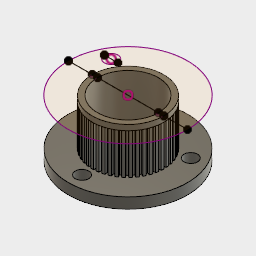
Slip Joint Gear v2 (Autodesk Fusion 360 design; units mm, degrees)
Autodesk Fusion 360 part; units mm, degrees
sketch "Sketch1" plane through (0, 0, 0) normal (0, 1, 0) x (1, 0, 0)
  circle A0 centre (0, 0) radius 22
  circle A1 centre (0, 0) radius 11.25
  line L0 (-0.0017, -22) -> (-0.0017, -19.5)
  circle A2 centre (-0.0017, -17) radius 2.5
  circle A3 centre (14.7233, 8.4986) radius 2.5
  circle A4 centre (-14.7216, 8.5014) radius 2.5
  dimension "d1" = 44
  dimension "d2" = 22.5
  dimension "d3" = 2.5
  dimension "d4" = 5
  dimension "d6" = 360
  measures "d1" diameter of A0
  measures "d2" diameter of A1
  measures "d3" distance of L0.start L0.end
  measures "d4" diameter of A2
extrude "Extrude1" add sketch "Sketch1" along normal blind 4
sketch "Sketch2" plane through (0, 4, 0) normal (0, 1, 0) x (-1, 0, 0)
  circle A0 centre (0, 0) radius 11.25
  circle A1 centre (14.7216, -8.5014) radius 2.5
  circle A2 centre (-14.7233, -8.4986) radius 2.5
  circle A3 centre (0.0017, 17) radius 2.5
  circle A4 centre (0, 0) radius 22
  circle A5 centre (0, 0) radius 12.25
  line L0 (0.0002, 13.25) -> (-0.5, 13.25)
  line L1 (-0.5, 13.25) -> (0.0002, 13.25)
  line L2 (0.0002, 13.25) -> (0.5, 13.25)
  line L3 (0.5, 13.25) -> (0.5, 12.2398)
  line L4 (-0.5, 13.25) -> (-0.5, 12.2398)
  line L5 (-2.3392, 13.0515) -> (-2.1986, 12.0511)
  line L6 (-1.8438, 13.1211) -> (-2.3392, 13.0515)
  line L7 (-1.8438, 13.1211) -> (-1.3489, 13.1906)
  line L8 (-1.3489, 13.1906) -> (-1.2083, 12.1903)
  line L9 (-4.1328, 12.5989) -> (-3.8544, 11.6278)
  line L10 (-3.652, 12.7368) -> (-4.1328, 12.5989)
  line L11 (-3.652, 12.7368) -> (-3.1716, 12.8745)
  line L12 (-3.1716, 12.8745) -> (-2.8931, 11.9035)
  line L13 (-5.846, 11.9011) -> (-5.4351, 10.9782)
  line L14 (-5.3891, 12.1046) -> (-5.846, 11.9011)
  line L15 (-5.3891, 12.1046) -> (-4.9325, 12.3078)
  line L16 (-4.9325, 12.3078) -> (-4.5216, 11.385)
  line L17 (-7.4455, 10.9717) -> (-6.9101, 10.115)
  line L18 (-7.0213, 11.2367) -> (-7.4455, 10.9717)
  line L19 (-7.0213, 11.2367) -> (-6.5974, 11.5016)
  line L20 (-6.5974, 11.5016) -> (-6.0621, 10.6449)
  line L21 (-8.9, 9.8287) -> (-8.2506, 9.0548)
  line L22 (-8.5168, 10.1502) -> (-8.9, 9.8287)
  line L23 (-8.5168, 10.1502) -> (-8.1339, 10.4715)
  line L24 (-8.1339, 10.4715) -> (-7.4846, 9.6976)
  line L25 (-10.1812, 8.4944) -> (-9.4305, 7.8184)
  line L26 (-9.8465, 8.8661) -> (-10.1812, 8.4944)
  line L27 (-9.8465, 8.8661) -> (-9.5121, 9.2376)
  line L28 (-9.5121, 9.2376) -> (-8.7614, 8.5616)
  line L29 (-11.2643, 6.9948) -> (-10.4268, 6.4299)
  line L30 (-10.9846, 7.4095) -> (-11.2643, 6.9948)
  line L31 (-10.9846, 7.4095) -> (-10.7052, 7.8238)
  line L32 (-10.7052, 7.8238) -> (-9.8677, 7.2589)
  line L33 (-12.1282, 5.359) -> (-11.2202, 4.9162)
  line L34 (-11.9089, 5.8086) -> (-12.1282, 5.359)
  line L35 (-11.9089, 5.8086) -> (-11.6898, 6.2578)
  line L36 (-11.6898, 6.2578) -> (-10.7819, 5.815)
  line L37 (-12.756, 3.6189) -> (-11.7952, 3.3068)
  line L38 (-12.6014, 4.0947) -> (-12.756, 3.6189)
  line L39 (-12.6014, 4.0947) -> (-12.447, 4.57)
  line L40 (-12.447, 4.57) -> (-11.4862, 4.2578)
  line L41 (-13.1355, 1.8084) -> (-12.1407, 1.633)
  line L42 (-13.0487, 2.301) -> (-13.1355, 1.8084)
  line L43 (-13.0487, 2.301) -> (-12.9619, 2.7932)
  line L44 (-12.9619, 2.7932) -> (-11.967, 2.6178)
  line L45 (-13.2594, -0.0373) -> (-12.2498, -0.0725)
  line L46 (-13.2419, 0.4626) -> (-13.2594, -0.0373)
  line L47 (-13.2419, 0.4626) -> (-13.2245, 0.9621)
  line L48 (-13.2245, 0.9621) -> (-12.2149, 0.9269)
  line L49 (-13.1252, -1.8823) -> (-12.1205, -1.7767)
  line L50 (-13.1774, -1.3848) -> (-13.1252, -1.8823)
  line L51 (-13.1774, -1.3848) -> (-13.2297, -0.8877)
  line L52 (-13.2297, -0.8877) -> (-12.225, -0.7821)
  line L53 (-12.7355, -3.6906) -> (-11.7553, -3.4462)
  line L54 (-12.8565, -3.2053) -> (-12.7355, -3.6906)
  line L55 (-12.8565, -3.2053) -> (-12.9774, -2.7203)
  line L56 (-12.9774, -2.7203) -> (-11.9972, -2.4759)
  line L57 (-12.0979, -5.4271) -> (-11.1612, -5.0487)
  line L58 (-12.2853, -4.9634) -> (-12.0979, -5.4271)
  line L59 (-12.2853, -4.9634) -> (-12.4725, -4.4999)
  line L60 (-12.4725, -4.4999) -> (-11.5358, -4.1215)
  line L61 (-11.2248, -7.058) -> (-10.35, -6.5529)
  line L62 (-11.4749, -6.6248) -> (-11.2248, -7.058)
  line L63 (-11.4749, -6.6248) -> (-11.7248, -6.192)
  line L64 (-11.7248, -6.192) -> (-10.85, -5.6869)
  line L65 (-10.1333, -8.5515) -> (-9.3373, -7.9296)
  line L66 (-10.4413, -8.1574) -> (-10.1333, -8.5515)
  line L67 (-10.4413, -8.1574) -> (-10.749, -7.7635)
  line L68 (-10.749, -7.7635) -> (-9.9529, -7.1416)
  line L69 (-8.8446, -9.8786) -> (-8.1428, -9.1519)
  line L70 (-9.2044, -9.5311) -> (-8.8446, -9.8786)
  line L71 (-9.2044, -9.5311) -> (-9.5639, -9.1839)
  line L72 (-9.5639, -9.1839) -> (-8.8621, -8.4572)
  line L73 (-7.3836, -11.0134) -> (-6.7899, -10.1961)
  line L74 (-7.7883, -10.7194) -> (-7.3836, -11.0134)
  line L75 (-7.7883, -10.7194) -> (-8.1927, -10.4256)
  line L76 (-8.1927, -10.4256) -> (-7.5989, -9.6083)
  line L77 (-5.779, -11.9338) -> (-5.3048, -11.0418)
  line L78 (-6.2207, -11.699) -> (-5.779, -11.9338)
  line L79 (-6.2207, -11.699) -> (-6.662, -11.4643)
  line L80 (-6.662, -11.4643) -> (-6.1877, -10.5724)
  line L81 (-4.0619, -12.6219) -> (-3.7164, -11.6727)
  line L82 (-4.532, -12.4509) -> (-4.0619, -12.6219)
  line L83 (-4.532, -12.4509) -> (-5.0016, -12.2799)
  line L84 (-5.0016, -12.2799) -> (-4.6561, -11.3306)
  line L85 (-2.2658, -13.0644) -> (-2.0557, -12.0763)
  line L86 (-2.755, -12.9604) -> (-2.2658, -13.0644)
  line L87 (-2.755, -12.9604) -> (-3.2439, -12.8565)
  line L88 (-3.2439, -12.8565) -> (-3.0339, -11.8684)
  line L89 (-0.4255, -13.2526) -> (-0.355, -12.2449)
  line L90 (-0.9245, -13.2177) -> (-0.4255, -13.2526)
  line L91 (-0.9245, -13.2177) -> (-1.4231, -13.1828)
  line L92 (-1.4231, -13.1828) -> (-1.3526, -12.1751)
  line L93 (1.4231, -13.1828) -> (1.3526, -12.1751)
  line L94 (0.9241, -13.2177) -> (1.4231, -13.1828)
  line L95 (0.9241, -13.2177) -> (0.4255, -13.2526)
  line L96 (0.4255, -13.2526) -> (0.355, -12.2449)
  line L97 (3.2439, -12.8565) -> (3.0339, -11.8684)
  line L98 (2.7546, -12.9605) -> (3.2439, -12.8565)
  line L99 (2.7546, -12.9605) -> (2.2658, -13.0644)
  line L100 (2.2658, -13.0644) -> (2.0557, -12.0763)
  line L101 (5.0016, -12.2799) -> (4.6561, -11.3306)
  line L102 (4.5316, -12.451) -> (5.0016, -12.2799)
  line L103 (4.5316, -12.451) -> (4.0619, -12.6219)
  line L104 (4.0619, -12.6219) -> (3.7164, -11.6727)
  line L105 (6.662, -11.4643) -> (6.1877, -10.5724)
  line L106 (6.2203, -11.6992) -> (6.662, -11.4643)
  line L107 (6.2203, -11.6992) -> (5.779, -11.9338)
  line L108 (5.779, -11.9338) -> (5.3048, -11.0418)
  line L109 (8.1927, -10.4256) -> (7.5989, -9.6083)
  line L110 (7.788, -10.7196) -> (8.1927, -10.4256)
  line L111 (7.788, -10.7196) -> (7.3836, -11.0134)
  line L112 (7.3836, -11.0134) -> (6.7899, -10.1961)
  line L113 (9.5639, -9.1839) -> (8.8621, -8.4572)
  line L114 (9.2041, -9.5314) -> (9.5639, -9.1839)
  line L115 (9.2041, -9.5314) -> (8.8446, -9.8786)
  line L116 (8.8446, -9.8786) -> (8.1428, -9.1519)
  line L117 (10.749, -7.7635) -> (9.9529, -7.1416)
  line L118 (10.441, -8.1577) -> (10.749, -7.7635)
  line L119 (10.441, -8.1577) -> (10.1333, -8.5515)
  line L120 (10.1333, -8.5515) -> (9.3373, -7.9296)
  line L121 (11.7248, -6.192) -> (10.85, -5.6869)
  line L122 (11.4747, -6.6252) -> (11.7248, -6.192)
  line L123 (11.4747, -6.6252) -> (11.2248, -7.058)
  line L124 (11.2248, -7.058) -> (10.35, -6.5529)
  line L125 (12.4725, -4.4999) -> (11.5358, -4.1215)
  line L126 (12.2851, -4.9637) -> (12.4725, -4.4999)
  line L127 (12.2851, -4.9637) -> (12.0979, -5.4271)
  line L128 (12.0979, -5.4271) -> (11.1612, -5.0487)
  line L129 (12.9774, -2.7203) -> (11.9972, -2.4759)
  line L130 (12.8564, -3.2057) -> (12.9774, -2.7203)
  line L131 (12.8564, -3.2057) -> (12.7355, -3.6906)
  line L132 (12.7355, -3.6906) -> (11.7553, -3.4462)
  line L133 (13.2297, -0.8877) -> (12.225, -0.7821)
  line L134 (13.1774, -1.3852) -> (13.2297, -0.8877)
  line L135 (13.1774, -1.3852) -> (13.1252, -1.8823)
  line L136 (13.1252, -1.8823) -> (12.1205, -1.7767)
  line L137 (13.2245, 0.9621) -> (12.2149, 0.9269)
  line L138 (13.2419, 0.4622) -> (13.2245, 0.9621)
  line L139 (13.2419, 0.4622) -> (13.2594, -0.0373)
  line L140 (13.2594, -0.0373) -> (12.2498, -0.0725)
  line L141 (12.9619, 2.7932) -> (11.967, 2.6178)
  line L142 (13.0487, 2.3006) -> (12.9619, 2.7932)
  line L143 (13.0487, 2.3006) -> (13.1355, 1.8084)
  line L144 (13.1355, 1.8084) -> (12.1407, 1.633)
  line L145 (12.447, 4.57) -> (11.4862, 4.2578)
  line L146 (12.6016, 4.0943) -> (12.447, 4.57)
  line L147 (12.6016, 4.0943) -> (12.756, 3.6189)
  line L148 (12.756, 3.6189) -> (11.7952, 3.3068)
  line L149 (11.6898, 6.2578) -> (10.7819, 5.815)
  line L150 (11.9091, 5.8082) -> (11.6898, 6.2578)
  line L151 (11.9091, 5.8082) -> (12.1282, 5.359)
  line L152 (12.1282, 5.359) -> (11.2202, 4.9162)
  line L153 (10.7052, 7.8238) -> (9.8677, 7.2589)
  line L154 (10.9849, 7.4091) -> (10.7052, 7.8238)
  line L155 (10.9849, 7.4091) -> (11.2643, 6.9948)
  line L156 (11.2643, 6.9948) -> (10.4268, 6.4299)
  line L157 (9.5121, 9.2376) -> (8.7614, 8.5616)
  line L158 (9.8468, 8.8658) -> (9.5121, 9.2376)
  line L159 (9.8468, 8.8658) -> (10.1812, 8.4944)
  line L160 (10.1812, 8.4944) -> (9.4305, 7.8184)
  line L161 (8.1339, 10.4715) -> (7.4846, 9.6976)
  line L162 (8.5171, 10.15) -> (8.1339, 10.4715)
  line L163 (8.5171, 10.15) -> (8.9, 9.8287)
  line L164 (8.9, 9.8287) -> (8.2506, 9.0548)
  line L165 (6.5974, 11.5016) -> (6.0621, 10.6449)
  line L166 (7.0216, 11.2365) -> (6.5974, 11.5016)
  line L167 (7.0216, 11.2365) -> (7.4455, 10.9717)
  line L168 (7.4455, 10.9717) -> (6.9101, 10.115)
  line L169 (4.9325, 12.3078) -> (4.5216, 11.385)
  line L170 (5.3894, 12.1044) -> (4.9325, 12.3078)
  line L171 (5.3894, 12.1044) -> (5.846, 11.9011)
  line L172 (5.846, 11.9011) -> (5.4351, 10.9782)
  line L173 (3.1716, 12.8745) -> (2.8931, 11.9035)
  line L174 (3.6524, 12.7367) -> (3.1716, 12.8745)
  line L175 (3.6524, 12.7367) -> (4.1328, 12.5989)
  line L176 (4.1328, 12.5989) -> (3.8544, 11.6278)
  line L177 (1.3489, 13.1906) -> (1.2083, 12.1903)
  line L178 (1.8442, 13.121) -> (1.3489, 13.1906)
  line L179 (1.8442, 13.121) -> (2.3392, 13.0515)
  line L180 (2.3392, 13.0515) -> (2.1986, 12.0511)
  dimension "d9" = 24.5
  dimension "d12" = 360
  measures "d9" diameter of A5
extrude "Extrude2" add sketch "Sketch2" along normal blind 15 contours A5 | A5 L137 L138 L139 L140 | A5 L141 L142 L143 L144 | A5 L133 L134 L135 L136 | A5 L145 L146 L147 L148 | A5 L129 L130 L131 L132 | A5 L149 L150 L151 L152 | A5 L125 L126 L127 L128 | A5 L153 L154 L155 L156 | A5 L121 L122 L123 L124 | A5 L157 L158 L159 L160 | A5 L117 L118 L119 L120 | A5 L161 L162 L163 L164 | A5 L113 L114 L115 L116 | A5 L165 L166 L167 L168 | A5 L109 L110 L111 L112 | A5 L169 L170 L171 L172 | A5 L105 L106 L107 L108 | A5 L173 L174 L175 L176 | A5 L101 L102 L103 L104 | A5 L177 L178 L179 L180 | A5 L97 L98 L99 L100 | A5 L0 L1 L2 L3 L4 | A5 L93 L94 L95 L96 | A5 L5 L6 L7 L8 | A5 L89 L90 L91 L92 | A5 L9 L10 L11 L12 | A5 L85 L86 L87 L88 | A5 L13 L14 L15 L16 | A5 L81 L82 L83 L84 | A5 L17 L18 L19 L20 | A5 L77 L78 L79 L80 | A5 L21 L22 L23 L24 | A5 L73 L74 L75 L76 | A5 L25 L26 L27 L28 | A5 L69 L70 L71 L72 | A5 L29 L30 L31 L32 | A5 L65 L66 L67 L68 | A5 L33 L34 L35 L36 | A5 L61 L62 L63 L64 | A5 L37 L38 L39 L40 | A5 L57 L58 L59 L60 | A5 L41 L42 L43 L44 | A5 L53 L54 L55 L56 | A5 L45 L46 L47 L48 | A5 L49 L50 L51 L52
sketch "Sketch3" plane through (0, 19, 0) normal (0, 1, 0) x (-1, 0, 0)
  circle A0 centre (0, 0) radius 11.25
  line L0 (2.3392, 13.0515) -> (1.3489, 13.1906)
  line L1 (1.3489, 13.1906) -> (1.2083, 12.1903)
  arc A1 (1.2083, 12.1903) -> (0.5, 12.2398) centre (0, 0) ccw
  line L2 (0.5, 12.2398) -> (0.5, 13.25)
  line L3 (0.5, 13.25) -> (-0.5, 13.25)
  line L4 (-0.5, 13.25) -> (-0.5, 12.2398)
  arc A2 (-0.5, 12.2398) -> (-1.2083, 12.1903) centre (0, 0) ccw
  line L5 (-1.2083, 12.1903) -> (-1.3489, 13.1906)
  line L6 (-1.3489, 13.1906) -> (-2.3392, 13.0515)
  line L7 (-2.3392, 13.0515) -> (-2.1986, 12.0511)
  arc A3 (-2.1986, 12.0511) -> (-2.8931, 11.9035) centre (0, 0) ccw
  line L8 (-2.8931, 11.9035) -> (-3.1716, 12.8745)
  line L9 (-3.1716, 12.8745) -> (-4.1328, 12.5989)
  line L10 (-4.1328, 12.5989) -> (-3.8544, 11.6278)
  arc A4 (-3.8544, 11.6278) -> (-4.5216, 11.385) centre (0, 0) ccw
  line L11 (-4.5216, 11.385) -> (-4.9325, 12.3078)
  line L12 (-4.9325, 12.3078) -> (-5.846, 11.9011)
  line L13 (-5.846, 11.9011) -> (-5.4351, 10.9782)
  arc A5 (-5.4351, 10.9782) -> (-6.0621, 10.6449) centre (0, 0) ccw
  line L14 (-6.0621, 10.6449) -> (-6.5974, 11.5016)
  line L15 (-6.5974, 11.5016) -> (-7.4455, 10.9717)
  line L16 (-7.4455, 10.9717) -> (-6.9101, 10.115)
  arc A6 (-6.9101, 10.115) -> (-7.4846, 9.6976) centre (0, 0) ccw
  line L17 (-7.4846, 9.6976) -> (-8.1339, 10.4715)
  line L18 (-8.1339, 10.4715) -> (-8.9, 9.8287)
  line L19 (-8.9, 9.8287) -> (-8.2506, 9.0548)
  arc A7 (-8.2506, 9.0548) -> (-8.7614, 8.5616) centre (0, 0) ccw
  line L20 (-8.7614, 8.5616) -> (-9.5121, 9.2376)
  line L21 (-9.5121, 9.2376) -> (-10.1812, 8.4944)
  line L22 (-10.1812, 8.4944) -> (-9.4305, 7.8184)
  arc A8 (-9.4305, 7.8184) -> (-9.8677, 7.2589) centre (0, 0) ccw
  line L23 (-9.8677, 7.2589) -> (-10.7052, 7.8238)
  line L24 (-10.7052, 7.8238) -> (-11.2643, 6.9948)
  line L25 (-11.2643, 6.9948) -> (-10.4268, 6.4299)
  arc A9 (-10.4268, 6.4299) -> (-10.7819, 5.815) centre (0, 0) ccw
  line L26 (-10.7819, 5.815) -> (-11.6898, 6.2578)
  line L27 (-11.6898, 6.2578) -> (-12.1282, 5.359)
  line L28 (-12.1282, 5.359) -> (-11.2202, 4.9162)
  arc A10 (-11.2202, 4.9162) -> (-11.4862, 4.2578) centre (0, 0) ccw
  line L29 (-11.4862, 4.2578) -> (-12.447, 4.57)
  line L30 (-12.447, 4.57) -> (-12.756, 3.6189)
  line L31 (-12.756, 3.6189) -> (-11.7952, 3.3068)
  arc A11 (-11.7952, 3.3068) -> (-11.967, 2.6178) centre (0, 0) ccw
  line L32 (-11.967, 2.6178) -> (-12.9619, 2.7932)
  line L33 (-12.9619, 2.7932) -> (-13.1355, 1.8084)
  line L34 (-13.1355, 1.8084) -> (-12.1407, 1.633)
  arc A12 (-12.1407, 1.633) -> (-12.2149, 0.9269) centre (0, 0) ccw
  line L35 (-12.2149, 0.9269) -> (-13.2245, 0.9621)
  line L36 (-13.2245, 0.9621) -> (-13.2594, -0.0373)
  line L37 (-13.2594, -0.0373) -> (-12.2498, -0.0725)
  arc A13 (-12.2498, -0.0725) -> (-12.225, -0.7821) centre (0, 0) ccw
  line L38 (-12.225, -0.7821) -> (-13.2297, -0.8877)
  line L39 (-13.2297, -0.8877) -> (-13.1252, -1.8823)
  line L40 (-13.1252, -1.8823) -> (-12.1205, -1.7767)
  arc A14 (-12.1205, -1.7767) -> (-11.9972, -2.4759) centre (0, 0) ccw
  line L41 (-11.9972, -2.4759) -> (-12.9774, -2.7203)
  line L42 (-12.9774, -2.7203) -> (-12.7355, -3.6906)
  line L43 (-12.7355, -3.6906) -> (-11.7553, -3.4462)
  arc A15 (-11.7553, -3.4462) -> (-11.5358, -4.1215) centre (0, 0) ccw
  line L44 (-11.5358, -4.1215) -> (-12.4725, -4.4999)
  line L45 (-12.4725, -4.4999) -> (-12.0979, -5.4271)
  line L46 (-12.0979, -5.4271) -> (-11.1612, -5.0487)
  arc A16 (-11.1612, -5.0487) -> (-10.85, -5.6869) centre (0, 0) ccw
  line L47 (-10.85, -5.6869) -> (-11.7248, -6.192)
  line L48 (-11.7248, -6.192) -> (-11.2248, -7.058)
  line L49 (-11.2248, -7.058) -> (-10.35, -6.5529)
  arc A17 (-10.35, -6.5529) -> (-9.9529, -7.1416) centre (0, 0) ccw
  line L50 (-9.9529, -7.1416) -> (-10.749, -7.7635)
  line L51 (-10.749, -7.7635) -> (-10.1333, -8.5515)
  line L52 (-10.1333, -8.5515) -> (-9.3373, -7.9296)
  arc A18 (-9.3373, -7.9296) -> (-8.8621, -8.4572) centre (0, 0) ccw
  line L53 (-8.8621, -8.4572) -> (-9.5639, -9.1839)
  line L54 (-9.5639, -9.1839) -> (-8.8446, -9.8786)
  line L55 (-8.8446, -9.8786) -> (-8.1428, -9.1519)
  arc A19 (-8.1428, -9.1519) -> (-7.5989, -9.6083) centre (0, 0) ccw
  line L56 (-7.5989, -9.6083) -> (-8.1927, -10.4256)
  line L57 (-8.1927, -10.4256) -> (-7.3836, -11.0134)
  line L58 (-7.3836, -11.0134) -> (-6.7899, -10.1961)
  arc A20 (-6.7899, -10.1961) -> (-6.1877, -10.5724) centre (0, 0) ccw
  line L59 (-6.1877, -10.5724) -> (-6.662, -11.4643)
  line L60 (-6.662, -11.4643) -> (-5.779, -11.9338)
  line L61 (-5.779, -11.9338) -> (-5.3048, -11.0418)
  arc A21 (-5.3048, -11.0418) -> (-4.6561, -11.3306) centre (0, 0) ccw
  line L62 (-4.6561, -11.3306) -> (-5.0016, -12.2799)
  line L63 (-5.0016, -12.2799) -> (-4.0619, -12.6219)
  line L64 (-4.0619, -12.6219) -> (-3.7164, -11.6727)
  arc A22 (-3.7164, -11.6727) -> (-3.0339, -11.8684) centre (0, 0) ccw
  line L65 (-3.0339, -11.8684) -> (-3.2439, -12.8565)
  line L66 (-3.2439, -12.8565) -> (-2.2658, -13.0644)
  line L67 (-2.2658, -13.0644) -> (-2.0557, -12.0763)
  arc A23 (-2.0557, -12.0763) -> (-1.3526, -12.1751) centre (0, 0) ccw
  line L68 (-1.3526, -12.1751) -> (-1.4231, -13.1828)
  line L69 (-1.4231, -13.1828) -> (-0.4255, -13.2526)
  line L70 (-0.4255, -13.2526) -> (-0.355, -12.2449)
  arc A24 (-0.355, -12.2449) -> (0.355, -12.2449) centre (0, 0) ccw
  line L71 (0.355, -12.2449) -> (0.4255, -13.2526)
  line L72 (0.4255, -13.2526) -> (1.4231, -13.1828)
  line L73 (1.4231, -13.1828) -> (1.3526, -12.1751)
  arc A25 (1.3526, -12.1751) -> (2.0557, -12.0763) centre (0, 0) ccw
  line L74 (2.0557, -12.0763) -> (2.2658, -13.0644)
  line L75 (2.2658, -13.0644) -> (3.2439, -12.8565)
  line L76 (3.2439, -12.8565) -> (3.0339, -11.8684)
  arc A26 (3.0339, -11.8684) -> (3.7164, -11.6727) centre (0, 0) ccw
  line L77 (3.7164, -11.6727) -> (4.0619, -12.6219)
  line L78 (4.0619, -12.6219) -> (5.0016, -12.2799)
  line L79 (5.0016, -12.2799) -> (4.6561, -11.3306)
  arc A27 (4.6561, -11.3306) -> (5.3048, -11.0418) centre (0, 0) ccw
  line L80 (5.3048, -11.0418) -> (5.779, -11.9338)
  line L81 (5.779, -11.9338) -> (6.662, -11.4643)
  line L82 (6.662, -11.4643) -> (6.1877, -10.5724)
  arc A28 (6.1877, -10.5724) -> (6.7899, -10.1961) centre (0, 0) ccw
  line L83 (6.7899, -10.1961) -> (7.3836, -11.0134)
  line L84 (7.3836, -11.0134) -> (8.1927, -10.4256)
  line L85 (8.1927, -10.4256) -> (7.5989, -9.6083)
  arc A29 (7.5989, -9.6083) -> (8.1428, -9.1519) centre (0, 0) ccw
  line L86 (8.1428, -9.1519) -> (8.8446, -9.8786)
  line L87 (8.8446, -9.8786) -> (9.5639, -9.1839)
  line L88 (9.5639, -9.1839) -> (8.8621, -8.4572)
  arc A30 (8.8621, -8.4572) -> (9.3373, -7.9296) centre (0, 0) ccw
  line L89 (9.3373, -7.9296) -> (10.1333, -8.5515)
  line L90 (10.1333, -8.5515) -> (10.749, -7.7635)
  line L91 (10.749, -7.7635) -> (9.9529, -7.1416)
  arc A31 (9.9529, -7.1416) -> (10.35, -6.5529) centre (0, 0) ccw
  line L92 (10.35, -6.5529) -> (11.2248, -7.058)
  line L93 (11.2248, -7.058) -> (11.7248, -6.192)
  line L94 (11.7248, -6.192) -> (10.85, -5.6869)
  arc A32 (10.85, -5.6869) -> (11.1612, -5.0487) centre (0, 0) ccw
  line L95 (11.1612, -5.0487) -> (12.0979, -5.4271)
  line L96 (12.0979, -5.4271) -> (12.4725, -4.4999)
  line L97 (12.4725, -4.4999) -> (11.5358, -4.1215)
  arc A33 (11.5358, -4.1215) -> (11.7553, -3.4462) centre (0, 0) ccw
  line L98 (11.7553, -3.4462) -> (12.7355, -3.6906)
  line L99 (12.7355, -3.6906) -> (12.9774, -2.7203)
  line L100 (12.9774, -2.7203) -> (11.9972, -2.4759)
  arc A34 (11.9972, -2.4759) -> (12.1205, -1.7767) centre (0, 0) ccw
  line L101 (12.1205, -1.7767) -> (13.1252, -1.8823)
  line L102 (13.1252, -1.8823) -> (13.2297, -0.8877)
  line L103 (13.2297, -0.8877) -> (12.225, -0.7821)
  arc A35 (12.225, -0.7821) -> (12.2498, -0.0725) centre (0, 0) ccw
  line L104 (12.2498, -0.0725) -> (13.2594, -0.0373)
  line L105 (13.2594, -0.0373) -> (13.2245, 0.9621)
  line L106 (13.2245, 0.9621) -> (12.2149, 0.9269)
  arc A36 (12.2149, 0.9269) -> (12.1407, 1.633) centre (0, 0) ccw
  line L107 (12.1407, 1.633) -> (13.1355, 1.8084)
  line L108 (13.1355, 1.8084) -> (12.9619, 2.7932)
  line L109 (12.9619, 2.7932) -> (11.967, 2.6178)
  arc A37 (11.967, 2.6178) -> (11.7952, 3.3068) centre (0, 0) ccw
  line L110 (11.7952, 3.3068) -> (12.756, 3.6189)
  line L111 (12.756, 3.6189) -> (12.447, 4.57)
  line L112 (12.447, 4.57) -> (11.4862, 4.2578)
  arc A38 (11.4862, 4.2578) -> (11.2202, 4.9162) centre (0, 0) ccw
  line L113 (11.2202, 4.9162) -> (12.1282, 5.359)
  line L114 (12.1282, 5.359) -> (11.6898, 6.2578)
  line L115 (11.6898, 6.2578) -> (10.7819, 5.815)
  arc A39 (10.7819, 5.815) -> (10.4268, 6.4299) centre (0, 0) ccw
  line L116 (10.4268, 6.4299) -> (11.2643, 6.9948)
  line L117 (11.2643, 6.9948) -> (10.7052, 7.8238)
  line L118 (10.7052, 7.8238) -> (9.8677, 7.2589)
  arc A40 (9.8677, 7.2589) -> (9.4305, 7.8184) centre (0, 0) ccw
  line L119 (9.4305, 7.8184) -> (10.1812, 8.4944)
  line L120 (10.1812, 8.4944) -> (9.5121, 9.2376)
  line L121 (9.5121, 9.2376) -> (8.7614, 8.5616)
  arc A41 (8.7614, 8.5616) -> (8.2506, 9.0548) centre (0, 0) ccw
  line L122 (8.2506, 9.0548) -> (8.9, 9.8287)
  line L123 (8.9, 9.8287) -> (8.1339, 10.4715)
  line L124 (8.1339, 10.4715) -> (7.4846, 9.6976)
  arc A42 (7.4846, 9.6976) -> (6.9101, 10.115) centre (0, 0) ccw
  line L125 (6.9101, 10.115) -> (7.4455, 10.9717)
  line L126 (7.4455, 10.9717) -> (6.5974, 11.5016)
  line L127 (6.5974, 11.5016) -> (6.0621, 10.6449)
  arc A43 (6.0621, 10.6449) -> (5.4351, 10.9782) centre (0, 0) ccw
  line L128 (5.4351, 10.9782) -> (5.846, 11.9011)
  line L129 (5.846, 11.9011) -> (4.9325, 12.3078)
  line L130 (4.9325, 12.3078) -> (4.5216, 11.385)
  arc A44 (4.5216, 11.385) -> (3.8544, 11.6278) centre (0, 0) ccw
  line L131 (3.8544, 11.6278) -> (4.1328, 12.5989)
  line L132 (4.1328, 12.5989) -> (3.1716, 12.8745)
  line L133 (3.1716, 12.8745) -> (2.8931, 11.9035)
  arc A45 (2.8931, 11.9035) -> (2.1986, 12.0511) centre (0, 0) ccw
  line L134 (2.1986, 12.0511) -> (2.3392, 13.0515)
  circle A46 centre (0, 0) radius 13.25
  circle A47 centre (0, 0) radius 11.25
extrude "Extrude3" add sketch "Sketch3" along normal blind 2 contours L1 A1 L2 L4 A2 L5 L7 A3 L8 L10 A4 L11 L13 A5 L14 L16 A6 L17 L19 A7 L20 L22 A8 L23 L25 A9 L26 L28 A10 L29 L31 A11 L32 L34 A12 L35 L37 A13 L38 L40 A14 L41 L43 A15 L44 L46 A16 L47 L49 A17 L50 L52 A18 L53 L55 A19 L56 L58 A20 L59 L61 A21 L62 L64 A22 L65 L67 A23 L68 L70 A24 L71 L73 A25 L74 L76 A26 L77 L79 A27 L80 L82 A28 L83 L85 A29 L86 L88 A30 L89 L91 A31 L92 L94 A32 L95 L97 A33 L98 L100 A34 L101 L103 A35 L104 L106 A36 L107 L109 A37 L110 L112 A38 L113 L115 A39 L116 L118 A40 L119 L121 A41 L122 L124 A42 L125 L127 A43 L128 L130 A44 L131 L133 A45 L134 A46 | L133 A45 L134 A46 | L1 A1 L2 A46 | L130 A44 L131 A46 | L4 A2 L5 A46 | L127 A43 L128 A46 | L7 A3 L8 A46 | L124 A42 L125 A46 | L10 A4 L11 A46 | L121 A41 L122 A46 | L13 A5 L14 A46 | L118 A40 L119 A46 | L16 A6 L17 A46 | L115 A39 L116 A46 | L19 A7 L20 A46 | L112 A38 L113 A46 | L22 A8 L23 A46 | L109 A37 L110 A46 | L25 A9 L26 A46 | L106 A36 L107 A46 | L28 A10 L29 A46 | L31 A11 L32 A46 | L103 A35 L104 A46 | L34 A12 L35 A46 | L100 A34 L101 A46 | L37 A13 L38 A46 | L97 A33 L98 A46 | L40 A14 L41 A46 | L94 A32 L95 A46 | L43 A15 L44 A46 | L91 A31 L92 A46 | L46 A16 L47 A46 | L88 A30 L89 A46 | L49 A17 L50 A46 | L85 A29 L86 A46 | L52 A18 L53 A46 | L82 A28 L83 A46 | L55 A19 L56 A46 | L79 A27 L80 A46 | L58 A20 L59 A46 | L76 A26 L77 A46 | L61 A21 L62 A46 | L73 A25 L74 A46 | L64 A22 L65 A46 | L70 A24 L71 A46 | L67 A23 L68 A46
sketch "Sketch4" plane through (0, 0, 0) normal (0, 0, 1) x (1, 0, 0)
  line L0 (-8.9, 4) -> (-8.9, 19)
  line L1 (-13.4277, 21) -> (13.25, 21)
  line L2 (22, 0) -> (-22, 0)
  line L3 (-22, 0) -> (22, 0)
  line L4 (-0.5, 19) -> (0.5, 19)
  line L5 (13.25, 21) -> (13.2419, 19)
  line L6 (13.25, 21) -> (-13.25, 21)
  line L7 (0.5, 4) -> (0.5, 19)
  line L8 (-0.5, 4) -> (-0.5, 19)
  point P0 (13.25, 21)
  point P1 (-22, 0)
  point P2 (-0.5, 19)
  point P3 (0.5, 19)
  point P4 (13.2419, 19)
  dimension "d17" = 2
  dimension "d18" = 26.5
  dimension "d19" = 44
  dimension "d20" = 1
  measures "d17" distance of P0 P4
  measures "d18" distance of P0 L6.end
  measures "d19" distance of L2.start P1
  measures "d20" distance of P2 P3
sketch "Sketch5" plane through (0, 21, 0) normal (0, 1, 0) x (-1, 0, 0)
  circle A0 centre (0, 0) radius 11.25
  circle A1 centre (0, 0) radius 13.25
  line L0 (11.25, 0) -> (-11.25, 0)
  circle A2 centre (14.7216, -8.5014) radius 2.5
  line L1 (17.2216, -8.5014) -> (12.2216, -8.5014)
  circle A3 centre (0, 0) radius 22
  line L2 (22, 0) -> (-22, 0)
  line L3 (13.2499, -0.0376) -> (-13.25, 0)
  point P0 (11.25, 0)
  point P1 (-11.25, 0)
  point P2 (17.2216, -8.5014)
  point P3 (22, 0)
  point P4 (13.2499, -0.0376)
  point P5 (-13.25, 0)
  dimension "d21" = 44
  dimension "d22" = 22.5
  dimension "d23" = 26.4999
  dimension "d24" = 5
  measures "d21" distance of P3 L2.end
  measures "d22" distance of P0 P1
  measures "d23" distance of P4 P5
  measures "d24" distance of P2 L1.end
